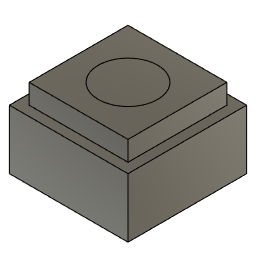
pambaram (Autodesk Fusion 360 design; units mm, degrees)
Autodesk Fusion 360 part; units mm, degrees
note: some values were not read from the file. Set by a fixed rule: which sketch regions a step uses.
sketch "Sketch1" plane through (0, 0, 0) normal (1, 0, 0) x (0, 1, 0)
  line L0 (0, 0) -> (0, 20)
  line L1 (0, 20) -> (3, 20)
  line L2 (3, 20) -> (15, 20)
  line L3 (15, 20) -> (15, 18.5)
  line L4 (2.4905, 2.2821) -> (3.1013, 9.2639)
  line L5 (7.906, 14.6253) -> (12.5862, 15.5578)
  arc A0 (7.906, 14.6253) -> (3.1013, 9.2639) centre (9.0785, 8.7409) ccw
  arc A1 (12.5862, 15.5578) -> (15, 18.5) centre (12, 18.5) ccw
  arc A2 (0, 0) -> (2.4905, 2.2821) centre (0, 2.5) ccw
  dimension "d2" = 15
  dimension "d14" = 6
  dimension "d15" = 5
  dimension "d16" = 3
  dimension "d17" = 20
  dimension "d18" = 1.5
  dimension "d20" = 5
  constraint vertical L0
  constraint perpendicular L0 L1
  constraint perpendicular L0 L2
  constraint perpendicular L2 L3
  constraint coincident L0 A2.centre
  constraint tangent L4 A2
  constraint tangent L4 A0
  constraint tangent L5 A0
  constraint tangent L5 A1
  constraint tangent L3 A1
  measures "d2" distance of L0 L3
  measures "d14" radius of A0
  measures "d15" diameter of A2
  measures "d16" radius of A1
  measures "d17" distance of L0.start L1
  measures "d18" distance of L2.end L3.end
  measures "d20" angle of L0 L4
revolve "Revolve2" add sketch "Sketch1" angle 360 about axis through (0, 0, 0) along (0, 0, 1) makes body 1
revolve "Revolve1" add sketch "Sketch1" angle 360 about axis through (0, 0, 0) along (0, 0, 1) separate body makes body 2
sketch "Sketch4" plane through (0, 0, 20) normal (0, 0, 1) x (-1, 0, 0)
  circle A0 centre (0, 0) radius 15
sketch "Sketch2" plane through (0, 0, 20) normal (0, 0, 1) x (-1, 0, 0)
  circle A0 centre (0, 0) radius 15
  line L0 (-25, -25) -> (25, -25)
  line L1 (25, -25) -> (25, 25)
  line L2 (25, 25) -> (-25, 25)
  line L3 (-25, 25) -> (-25, -25)
  line L4 (-25, -25) -> (25, 25) construction
  line L5 (25, -25) -> (-25, 25) construction
  dimension "d4" = 50
  dimension "d5" = 50
  constraint horizontal L0
  constraint perpendicular L0 L1
  constraint parallel L0 L2
  constraint parallel L1 L3
  constraint coincident L4 A0.centre
  constraint coincident L5 A0.centre
  constraint coincident A0.centre origin
  measures "d4" distance of L1.end L2.end
  measures "d5" distance of L0.end L1.end
extrude "Extrude1" add sketch "Sketch2" against normal blind 25 separate body contours A0 | L0 L1 L2 L3 makes body 3
combine "Combine1" operation cut target body 3 tool bodies 2 keep tools
sketch "Sketch3" plane through (0, 0, 20) normal (0, 0, 1) x (-1, 0, 0)
  circle A0 centre (0, 0) radius 15
  line L0 (-25, 25) -> (-25, -25)
  line L1 (-25, -25) -> (25, -25)
  line L2 (25, -25) -> (25, 25)
  line L3 (25, 25) -> (-25, 25)
  circle A1 centre (0, 0) radius 15
  line L4 (-30, -30) -> (30, -30)
  line L5 (30, -30) -> (30, 30)
  line L6 (30, 30) -> (-30, 30)
  line L7 (-30, 30) -> (-30, -30)
  line L8 (-30, -30) -> (30, 30) construction
  line L9 (30, -30) -> (-30, 30) construction
  dimension "d8" = 5
  constraint horizontal L4
  constraint perpendicular L4 L5
  constraint parallel L4 L6
  constraint parallel L5 L7
  constraint coincident L8 A0.centre
  constraint coincident L9 A0.centre
  constraint coincident A0.centre A1.centre
  constraint equal L4 L5
  measures "d8" distance of L1 L4
extrude "Extrude2" add sketch "Sketch3" along normal blind 5 and the other way blind 25 separate body contours A0 A1 | L0 L1 L2 L3 | L4 L5 L6 L7 makes body 4
combine "Combine2" operation cut target body 4 tool bodies 3 keep tools
move_body "Move2" bodies 4 to x (-1, 0, 0) y (0, 1, 0) z (0, 0, -1) at (0, 0, 5)
